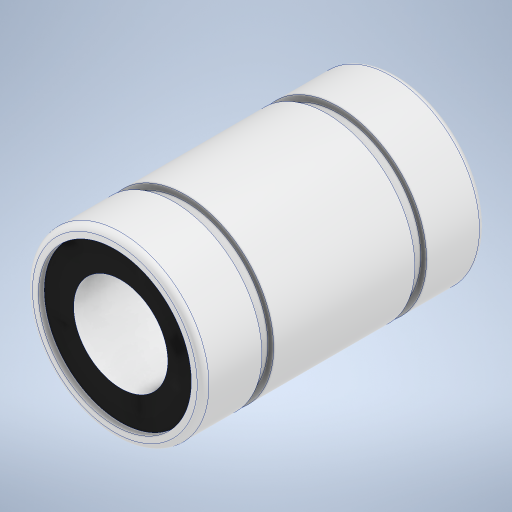
# Autodesk Inventor part: berring
Saved by Autodesk Inventor 2023 (Build 270158000, 158)
## iProperties
Created: 2023-07-16
Part Number: berring
Material: Aluminum 6061
Document SubType Name: Modeling
Designer: checo
Density: 2.7 g/cm^3
Appearance: Aluminum - Flat
Author: checo
Autodesk Inventor part; units mm, degrees
ref_plane "YZ Plane" through (0, 0, 0) normal (1, 0, 0) x (0, 1, 0)
ref_plane "XZ Plane" through (0, 0, 0) normal (0, 1, 0) x (-1, 0, 0)
ref_plane "XY Plane" through (0, 0, 0) normal (0, 0, 1) x (1, 0, 0)
sketch "Sketch1" plane through (0, 0, 0) normal (0, 0, 1) x (1, 0, 0)
  circle A0 centre (0, 0) radius 4
  circle A1 centre (0, 0) radius 7.5
  dimension "d2" = 8
  dimension "d3" = 15
  constraints: 2 centre point, 2 coincident
  measures "d2" diameter of A0
  measures "d3" diameter of A1
extrude "Extrusion1" add sketch "Sketch1" along normal blind 24
fillet "Fillet1" radius 0.5 2 edges at (-7.5, 0, 24) (-7.5, 0, 0)
sketch "Sketch2" plane through (0, 0, 0) normal (1, 0, 0) x (0, 1, 0)
  arc A0 (7, 0) -> (7.5, 0.5) centre (7, 0.5) ccw projected
  line L0 (7, 0) -> (4, 0) projected
  line L1 (4, 0) -> (4, 24) projected
  line L2 (4, 24) -> (7, 24) projected
  arc A1 (7.5, 23.5) -> (7, 24) centre (7, 23.5) ccw projected
  line L3 (7.5, 23.5) -> (7.5, 0.5) projected
  arc A2 (-7.5, 0.5) -> (-7, 0) centre (-7, 0.5) ccw projected
  line L4 (-7.5, 0.5) -> (-7.5, 23.5) projected
  arc A3 (-7, 24) -> (-7.5, 23.5) centre (-7, 23.5) ccw projected
  line L5 (-7, 24) -> (-4, 24) projected
  line L6 (-4, 24) -> (-4, 0) projected
  line L7 (-4, 0) -> (-7, 0) projected
  line L8 (7.5, 0.5) -> (7.5, 23.5) projected
  line L9 (7.5, 19) -> (7, 19)
  line L10 (7, 19) -> (7, 18)
  line L11 (7, 18) -> (7.5, 18)
  line L12 (7.5, 12) -> (4, 12) construction
  line L13 (7.5, 5) -> (7, 5)
  line L14 (7, 5) -> (7, 6)
  line L15 (7, 6) -> (7.5, 6)
  line L16 (-4, 24) -> (4, 24) construction
  line L17 (0, 24) -> (0, 0) construction
  dimension "d5" = 5
  dimension "d6" = 1
  dimension "d7" = 0.5
  constraints: 16 end point, 4 symmetric about line, 3 midpoint, 2 perpendicular, 2 point on line, 1 horizontal, 1 vertical
  measures "d5" distance between parallel lines of L9 L2
  measures "d6" distance of L9.end L10.end
  measures "d7" distance between parallel lines of L3 L10
revolve "Revolution1" cut sketch "Sketch2" angle 360 about axis through (0, 0, 24) along (0, 0, -1) contours L13 L14 L15 L3 | L11 L10 L9 L3
sketch "Sketch3" plane through (0, 0, 24) normal (0, 0, 1) x (1, 0, 0)
  circle A0 centre (0, 0) radius 6.5
  circle A1 centre (0, 0) radius 7.5 projected
  dimension "d9" = 1
  constraints: 1 centre point, 1 coincident
  measures "d9" radial gap between concentric circles of A1 A0
extrude "Extrusion2" cut sketch "Sketch3" against normal blind 0.5 contours A0
extrude "Extrusion3" cut sketch "Sketch3" along normal blind 0.5 from surface at -24 contours A0
body "Solid1"
